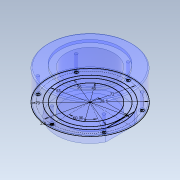
# Autodesk Inventor part: motor_simplified
Saved by Autodesk Inventor 2020 (Build 240168000, 168)
## iProperties
Created: 2021-02-18
Part Number: motor_simplified
Material: Generic
Document SubType Name: Modeling
Designer: DELL
Density: 1 g/cm^3
Appearance: Clear - Blue
Author: DELL
Autodesk Inventor part; units mm, degrees
ref_plane "YZ Plane" through (0, 0, 0) normal (1, 0, 0) x (0, 1, 0)
ref_plane "XZ Plane" through (0, 0, 0) normal (0, 1, 0) x (-1, 0, 0)
ref_plane "XY Plane" through (0, 0, 0) normal (0, 0, 1) x (1, 0, 0)
sketch "Sketch1" plane through (0, 0, 0) normal (0, 1, 0) x (-1, 0, 0)
  circle A0 centre (0, 0) radius 39.5
  circle A1 centre (0, 0) radius 31.5
  circle A2 centre (0, 0) radius 28
  line L0 (-28.5, 13.4164) -> (-28.5, -13.4164)
  circle A3 centre (0, 0) radius 36 construction
  line L1 (0, 39.5) -> (0, 0) construction
  line L2 (0, 0) -> (-34.208, 19.75) construction
  circle A4 centre (0, 36) radius 1.4
  circle A5 centre (-31.1769, 18) radius 1.4
  line L3 (0, 0) -> (-39.5, 0) construction
  circle A6 centre (31.1769, 18) radius 1.4
  circle A7 centre (0, -36) radius 1.4
  circle A8 centre (-31.1769, -18) radius 1.4
  circle A9 centre (31.1769, -18) radius 1.4
  circle A10 centre (0, 0) radius 22.5
  dimension "d0" = 79
  dimension "d1" = 63
  dimension "d2" = 56
  dimension "d6" = 28.5
  dimension "d11" = 72
  dimension "d12" = 2.8
  dimension "d13" = 60
  dimension "d19" = 45
  constraints: 11 centre point, 8 end point, 7 point on circle, 5 coincident, 4 symmetric about line, 2 point on line, 2 vertical, 1 equal radius, 1 horizontal, 4 other
  measures "d0" diameter of A0
  measures "d1" diameter of A1
  measures "d2" diameter of A2
  measures "d6" distance from line of point (0, 0) L0
  measures "d11" diameter of A3
  measures "d12" diameter of A4
  measures "d13" angle of L1 L2
  measures "d19" diameter of A10
extrude "Extrusion1" add sketch "Sketch1" along normal blind 29 contours A0 | A1 L0 | L0 A1 | A2 | A4 | A5 | A6 | A7 | A8 | A9 | A10
extrude "Extrusion2" add sketch "Sketch1" against normal blind 11.5 contours A1 L0 | A2 | A10 picked at (29.747, 4.7866)
extrude "Extrusion3" add sketch "Sketch1" along normal blind 2.5 from surface at 29 contours A2 | A10
extrude "Extrusion4" cut sketch "Sketch1" along normal blind 15 contours A4 | A5 | A6 | A7 | A8 | A9
chamfer "Chamfer1" distance 1 angle 45 6 edges at (1.4, 0, -36) (-29.7769, 0, -18) (-29.7769, 0, 18) (32.5769, 0, -18) (32.5769, 0, 18) (1.4, 0, 36)
extrude "Extrusion5" cut sketch "Sketch1" along normal blind 29 and the other way blind 8.25 contours A10
fillet "Fillet1" radius 1 1 edges at (39.5, 0, 0)
fillet "Fillet2" radius 1 1 edges at (39.5, 29, 0)
body "Solid1"
